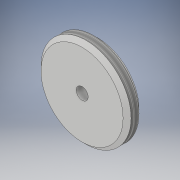
# Autodesk Inventor part: new_encoder
Saved by Autodesk Inventor 2019 (Build 230136000, 136)
## iProperties
Created: 2020-02-17
Part Number: new_encoder
Material: Generic
Document SubType Name: Modeling
Designer: Prajwal
Density: 1 g/cm^3
Appearance: Default
Author: Prajwal
Autodesk Inventor part; units mm, degrees
ref_plane "YZ Plane" through (0, 0, 0) normal (1, 0, 0) x (0, 1, 0)
ref_plane "XZ Plane" through (0, 0, 0) normal (0, 1, 0) x (-1, 0, 0)
ref_plane "XY Plane" through (0, 0, 0) normal (0, 0, 1) x (1, 0, 0)
sketch "Sketch1" plane through (0, 0, 0) normal (0, 0, 1) x (1, 0, 0)
  circle A0 centre (0, 0) radius 56.5
  dimension "d0" = 113
  constraints: 1 centre point, 1 coincident
  measures "d0" diameter of A0
extrude "Extrusion1" add sketch "Sketch1" along normal blind 20
thread "Thread1" size "M115x6" class "6g" standard "ANSI Metric M Profile" full length
chamfer "Chamfer1" distance 5 angle 45 2 edges at (-56.5, 0, 20) (-56.5, 0, 0)
sketch "Sketch2" plane through (0, 0, 20) normal (0, 0, 1) x (1, 0, 0)
  point P0 (0, 0)
  point P1 (0.2077, 1.3498)
hole "Hole1" at (0.2077, 1.3498, 20) direction (0, 0, -1) diameter 15 depth 20 tip angle 118
body "Solid1"
